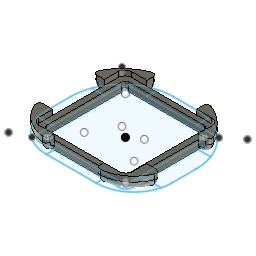
seria_case_adapter_small v1 (Autodesk Fusion 360 design; units mm, degrees)
Autodesk Fusion 360 part; units mm, degrees
sketch "スケッチ1" plane through (0, 0, 0) normal (0, 0, 1) x (1, 0, 0)
  line L0 (23.3, -27) -> (-23.3, -27)
  line L1 (-27.3, -23) -> (-27.3, 23)
  line L2 (-23.3, 27) -> (23.3, 27)
  line L3 (27.3, 23) -> (27.3, -23)
  arc A0 (-23.3, 27) -> (-27.3, 23) centre (-23.3, 23) ccw
  arc A1 (27.3, 23) -> (23.3, 27) centre (23.3, 23) ccw
  arc A2 (23.3, -27) -> (27.3, -23) centre (23.3, -23) ccw
  arc A3 (-27.3, -23) -> (-23.3, -27) centre (-23.3, -23) ccw
  line L4 (14.5, -31.5) -> (-14.5, -31.5)
  line L5 (-36.5, -9.5) -> (-36.5, 4.5)
  line L6 (-6.5, 34.5) -> (6.5, 34.5)
  line L7 (36.5, 4.5) -> (36.5, -9.5)
  arc A4 (-6.5, 34.5) -> (-36.5, 4.5) centre (-6.5, 4.5) ccw
  arc A5 (36.5, 4.5) -> (6.5, 34.5) centre (6.5, 4.5) ccw
  arc A6 (-36.5, -9.5) -> (-14.5, -31.5) centre (-14.5, -9.5) ccw
  arc A7 (14.5, -31.5) -> (36.5, -9.5) centre (14.5, -9.5) ccw
  line L8 (-34.6025, 15) -> (-27.3, 15)
  line L9 (27.3, 15) -> (34.6025, 15)
  line L10 (14.5, 33.4137) -> (14.5, 27)
  line L11 (14.5, -27) -> (14.5, -31.5)
  line L12 (-14.5, -31.5) -> (-14.5, -27)
  line L13 (-14.5, 27) -> (-14.5, 33.4137)
  line L14 (35.8014, -15) -> (27.3, -15)
  line L15 (-27.3, -15) -> (-35.8014, -15)
  line L16 (-22, 24) -> (22, 24)
  line L17 (24, 22) -> (24, -22)
  line L18 (22, -24) -> (-22, -24)
  line L19 (-24, -22) -> (-24, 22)
  arc A8 (-22, 24) -> (-24, 22) centre (-22, 22) ccw
  arc A9 (24, 22) -> (22, 24) centre (22, 22) ccw
  arc A10 (22, -24) -> (24, -22) centre (22, -22) ccw
  arc A11 (-24, -22) -> (-22, -24) centre (-22, -22) ccw
  point P0 (-27.3, -27)
  point P1 (-27.3, 27)
  point P2 (27.3, 27)
  point P3 (-36.5, -31.5)
  point P4 (-36.5, 34.5)
  point P5 (36.5, 34.5)
  dimension "d1" = 54.6
  dimension "d2" = 54
  dimension "d3" = 4
  dimension "d4" = 73
  dimension "d5" = 66
  dimension "d6" = 30
  dimension "d7" = 30
  dimension "d8" = 22
  dimension "d9" = 2
  constraint horizontal L0
  constraint perpendicular L0 L1
  constraint parallel L0 L2
  constraint parallel L1 L3
  constraint coincident P1 L1
  constraint coincident P1 L2
  constraint tangent L1 A0
  constraint tangent L2 A0
  constraint coincident P2 L2
  constraint coincident P2 L3
  constraint tangent L2 A1
  constraint tangent L3 A1
  constraint equal A0 A1
  constraint tangent L0 A2
  constraint tangent L3 A2
  constraint equal A0 A2
  constraint coincident P0 L0
  constraint coincident P0 L1
  constraint tangent L0 A3
  constraint tangent L1 A3
  constraint equal A0 A3
  constraint horizontal L4
  constraint perpendicular L4 L5
  constraint parallel L4 L6
  constraint parallel L5 L7
  constraint coincident P4 L5
  constraint coincident P4 L6
  constraint tangent L5 A4
  constraint tangent L6 A4
  constraint coincident P5 L6
  constraint coincident P5 L7
  constraint tangent L6 A5
  constraint tangent L7 A5
  constraint coincident P3 L4
  constraint coincident P3 L5
  constraint tangent L4 A6
  constraint tangent L5 A6
  constraint tangent L4 A7
  constraint tangent L7 A7
  constraint equal A6 A7
  constraint horizontal L8
  constraint horizontal L14
  constraint vertical L10
  constraint vertical L12
  constraint coincident A4 L13.end
  constraint coincident A5 L10.start
  constraint coincident A4 L8.start
  constraint coincident A6 L15.end
  constraint coincident A5 L9.end
  constraint coincident A7 L14.start
  constraint coincident L1 L8.end
  constraint collinear L8 L9
  constraint coincident L3 L9.start
  constraint coincident L2 L10.end
  constraint collinear L10 L11
  constraint coincident L2 L13.start
  constraint collinear L12 L13
  constraint coincident L1 L15.start
  constraint collinear L14 L15
  constraint coincident L3 L14.end
  constraint coincident L0 L12.end
  constraint coincident L0 L11.start
  constraint horizontal L16
  constraint vertical L17
  constraint horizontal L18
  constraint vertical L19
  constraint tangent L16 A8
  constraint tangent L19 A8
  constraint tangent L16 A9
  constraint tangent L17 A9
  constraint equal A8 A9
  constraint tangent L17 A10
  constraint tangent L18 A10
  constraint equal A8 A10
  constraint tangent L18 A11
  constraint tangent L19 A11
  constraint equal A8 A11
  measures "d1" distance of P1 P2
  measures "d2" distance of P0 P1
  measures "d3" radius of A0
  measures "d4" distance of P4 P5
  measures "d5" distance of P3 P4
  measures "d6" radius of A4
  measures "d7" radius of A5
  measures "d8" radius of A6
  measures "d9" radius of A8
extrude "押し出し1" add sketch "スケッチ1" along normal blind 5 contours L0 L1 L2 L3 A0 A1 A2 A3
extrude "押し出し2" add sketch "スケッチ1" along normal blind 8 contours L0 L3 A2 A7 L11 L14 | L0 L1 A3 A6 L12 L15 | L2 L3 A1 A5 L9 L10 | L1 L2 A0 A4 L8 L13
fillet "フィレット3" radius 5 2 edges at (26.7636, 26.6221, 0) (-26.7636, 26.6221, 0)
extrude "押し出し3" cut 1 faces at (4.8333, -27, 3.3333) along direction (0, 1, 0) blind 1
fillet "フィレット4" radius 5 2 edges at (-27.9722, -26.8925, 0) (27.9722, -26.8925, 0)
fillet "フィレット5" radius 2 24 edges at (14.5, -31.5, 6.5) (14.5, -30.0355, 1.4645) (14.5, -26.25, 0) (-14.5, -26.25, 0) (-14.5, -30.0355, 1.4645) (-14.5, -31.5, 6.5) (-35.8014, -15, 6.5) (-34.244, -15, 1.4252) (-28.9429, -15, 0) (-28.2441, 15, 0) (-32.9544, 15, 1.3926) (-34.6025, 15, 6.5) (-14.5, 33.4137, 6.5) (-14.5, 31.8492, 1.4247) (-14.5, 27.5927, 0) (14.5, 27.5927, 0) (14.5, 31.8492, 1.4247) (14.5, 33.4137, 6.5) (34.6025, 15, 6.5) (32.9544, 15, 1.3926) (28.2441, 15, 0) (28.9429, -15, 0) (34.244, -15, 1.4252) (35.8014, -15, 6.5)
extrude "押し出し4" add 1 faces at (4.8333, -26, 3) along direction (0, -1, 0) blind 1
